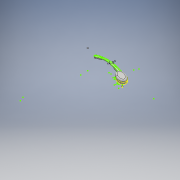
# Autodesk Inventor part: InnerPod
Saved by Autodesk Inventor 2016 (Build 200138000, 138)
## iProperties
Created: 2015-06-15
Part Number: InnerPod
Material: Generic
Document SubType Name: Modeling
Designer: Erin
Density: 1 g/cm^3
Appearance: Default
Author: Erin
Autodesk Inventor part; units mm, degrees
ref_plane "YZ Plane" through (0, 0, 0) normal (1, 0, 0) x (0, 1, 0)
sketch "Sketch1" plane through (0, 0, 0) normal (0, 0, 1) x (1, 0, 0)
  line L0 (0, -23.0647) -> (0, 59.7901) construction
  ellipse E0 centre (-14.0004, 12.1) end of major axis (-23.0535, 16.1357) minor radius 4.9157
  arc A0 (-24.1451, 19.8468) -> (-50.54, 25.9478) centre (-70.9085, -122.3194) ccw
  arc A1 (-29.3261, 18.5387) -> (-51.8244, 24.0854) centre (-73.9314, -113.9855) ccw
  arc A2 (-31.8925, 10.9139) -> (-44.4376, 12.262) centre (-55.0181, -145.2384) ccw
  arc A3 (-31.8925, 10.9139) -> (-26.6229, 7.7379) centre (-17.4265, 28.9559) ccw
  arc A4 (-24.9409, 14.9636) -> (-22.1909, 12.262) centre (-19.0136, 18.2468) ccw
  arc A5 (-26.6229, 7.7379) -> (-13.0654, 6.572) centre (-17.1508, 38.4743) ccw
  arc A6 (-24.9409, 14.9636) -> (-29.3261, 18.5387) centre (-31.8925, 10.9139) ccw
  arc A7 (-24.1451, 19.8468) -> (-17.2584, 18.0641) centre (-13.8815, 45.3013) ccw
  arc A8 (-50.54, 25.9478) -> (-75.3937, 22.2872) centre (-55.9595, -23.4584) ccw
  arc A9 (-75.3937, 22.2872) -> (-71.6688, 21.067) centre (-73.3522, 22.2238) ccw
  arc A10 (-51.8244, 24.0854) -> (-71.6688, 21.067) centre (-57.2432, -7.0315) ccw
  arc A11 (-75.3937, 22.2872) -> (-90.8007, 8.3693) centre (-63.623, -6.2295) ccw
  arc A12 (-44.4376, 12.262) -> (-65.1692, 5.2101) centre (-38.8966, -38.0273) ccw
  arc A13 (-69.6317, 5.2101) -> (-65.1692, 5.2101) centre (-67.4004, 17.1946) ccw
  arc A14 (-69.6317, 5.2101) -> (-86.7264, 2.9791) centre (-74.6345, -23.0647) ccw
  arc A15 (-91.0496, 2.5661) -> (-86.7264, 2.9791) centre (-89.7462, 11.7565) ccw
  arc A16 (-90.8007, 8.3693) -> (-91.0496, 2.5661) centre (-84.9194, 5.2101) ccw
  ellipse E1 centre (-14.0004, 12.1) end of major axis (-23.7436, 16.5326) minor radius 5.7074
  ellipse E2 centre (-14.0004, 12.1) end of major axis (-25.1676, 17.1231) minor radius 7.2205
  line L1 (-14.1688, 17.4082) -> (7.9431, 10.5495) construction
  line L2 (-13.9565, 18.1799) -> (8.2098, 11.3044) construction
  line L3 (-5.6332, 7.1546) -> (-15.3689, -1.2851) construction
  line L4 (-5.0965, 6.5612) -> (-14.2425, -1.3674) construction
  line L5 (-4.0088, 5.519) -> (-10.8447, -0.4071) construction
  line L6 (-13.3724, 19.5692) -> (7.8363, 12.9908) construction
  line L7 (-9.6767, 18.0114) -> (-18.3242, 6.1886)
  arc A17 (-50.3962, 27.1116) -> (-75.8521, 23.3664) centre (-55.9595, -23.4584) ccw
  arc A18 (-24.0317, 20.2324) -> (-17.2091, 18.461) centre (-13.8815, 45.3013) ccw
  arc A19 (-76.7002, 22.3279) -> (-70.8185, 20.0327) centre (-73.3522, 22.2238) ccw
  arc A20 (-52.04, 22.7961) -> (-70.8185, 20.0327) centre (-57.2432, -7.0315) ccw
  arc A21 (-25.2887, 14.7659) -> (-29.4537, 18.1596) centre (-31.8925, 10.9139) ccw
  arc A22 (-25.2887, 14.7659) -> (-22.3785, 11.9087) centre (-19.0136, 18.2468) ccw
  arc A23 (-26.8006, 7.3741) -> (-13.0146, 6.1752) centre (-17.1508, 38.4743) ccw
  arc A24 (-32.3718, 9.8038) -> (-44.4122, 11.0896) centre (-55.0181, -145.2384) ccw
  arc A25 (-44.4122, 11.0896) -> (-64.7397, 4.1038) centre (-38.8966, -38.0273) ccw
  arc A26 (-69.8402, 4.0608) -> (-64.7397, 4.1038) centre (-67.4004, 17.1946) ccw
  arc A27 (-69.8402, 4.0608) -> (-86.2871, 1.8952) centre (-74.6345, -23.0647) ccw
  arc A28 (-91.8404, 1.5181) -> (-86.2871, 1.8952) centre (-89.7462, 11.7565) ccw
  arc A29 (-91.8297, 8.9221) -> (-91.8404, 1.5181) centre (-84.9194, 5.2101) ccw
  arc A30 (-75.8393, 23.3669) -> (-91.8297, 8.9221) centre (-63.623, -6.2295) ccw
  line L8 (22.4734, 0) -> (-109.3623, 0) construction
  line L9 (0, 0) -> (-2, 0)
  line L10 (-2, 0) -> (-2, 2)
  line L11 (-2, 2) -> (0, 2)
  line L12 (0, 2) -> (0, 0)
  line L13 (-97, 32) -> (-95, 32)
  line L14 (-95, 32) -> (-95, 30)
  line L15 (-95, 30) -> (-97, 30)
  line L16 (-97, 30) -> (-97, 32)
  dimension "d9" = 0.8
  dimension "d11" = 0.8
  dimension "d14" = 1.5
  dimension "d16" = 1.5
  dimension "d21" = 0.4
  dimension "d22" = 0.4
  dimension "d23" = 0.4
  dimension "d64" = 2
  dimension "d65" = 2
  dimension "d66" = 2
  dimension "d67" = 2
  dimension "d68" = 30
  dimension "d69" = 95
  constraints: 62 point on circle, 34 end point, 31 centre point, 7 parallel, 4 horizontal, 2 perpendicular, 2 vertical, 35 other
  measures "d9" distance between parallel lines of L1 L2
  measures "d11" distance between parallel lines of L4 L3
  measures "d14" distance between parallel lines of L4 L5
  measures "d16" distance between parallel lines of L2 L6
  measures "d21" radial gap between concentric circles of A7 A18
  measures "d22" radial gap between concentric circles of A4 A22
  measures "d23" radial gap between concentric circles of A5 A23
  measures "d64" distance of L10.end L11.end
  measures "d65" distance of L9.end L10.end
  measures "d66" distance of L14.end L15.end
  measures "d67" distance of L13.end L14.end
  measures "d68" distance between parallel lines of L15 L8
  measures "d69" distance between parallel lines of L14 L0
extrude "Extrusion4" add sketch "Sketch1" along normal blind 6.4 contours E0 L7 | E0 A4 E1 A7 | E0 L7 E1 A4 | A7 E1 L7 E0 | L7 E0 | E0 A5 E1 L7 | E1 A22 A21 E2 A6 A4 | A4 A6 E2 A7 E1 | L7 E1 A5 E0 | A7 E2 A18 E1 | L7 A5 E2 A21 A22 E1 | E1 A5 L7 | L7 E2 A23 E1 | E1 A18 E2 L7 | E1 A23 E2 L7 A5 | L7 E2 A5
extrude "Extrusion5" cut sketch "Sketch1" along normal blind 5.4 contours E0 L7 | E0 A4 E1 A7 | E0 L7 E1 A4 | A7 E1 L7 E0 | L7 E0 | E0 A5 E1 L7 | L7 E1 A5 E0
sketch "Sketch3" plane through (0, 0, 0) normal (0, 0, 1) x (1, 0, 0)
  arc A0 (-22.4417, 19.646) -> (-19.6295, 18.8734) centre (-13.8815, 45.3013) ccw
  arc A1 (-25.2887, 14.7659) -> (-23.0979, 12.3467) centre (-19.0136, 18.2468) ccw
  arc A2 (-25.2887, 14.7659) -> (-25.5583, 15.1947) centre (-31.8925, 10.9139) ccw
  arc A3 (-17.8075, 5.9181) -> (-14.1373, 6.0512) centre (-17.1508, 38.4743) ccw
  ellipse E0 centre (-14.0004, 12.1) end of major axis (-25.1676, 17.1231) minor radius 7.2205 projected
  ellipse E1 centre (-14.0004, 12.1) end of major axis (-23.7436, 16.5326) minor radius 5.7074 projected
  ellipse E2 centre (-14.0004, 12.1) end of major axis (-4.2573, 7.6674) minor radius 5.7074 projected
  line L0 (-14.1321, 6.0475) -> (-18.4635, 9.206)
  line L1 (-18.4635, 9.206) -> (-23.0991, 12.3388)
  ellipse E3 centre (-14.0004, 12.1) end of major axis (-25.1676, 17.1231) minor radius 7.2205 projected
  line L2 (-17.805, 5.9169) -> (-22.6057, 8.0763)
  line L3 (-22.6057, 8.0763) -> (-25.7428, 12.7137)
  line L4 (-25.7428, 12.7137) -> (-25.5519, 15.1307)
  line L5 (-25.5519, 15.1307) -> (-25.9604, 19.264)
  line L6 (-25.9604, 19.264) -> (-22.42, 19.6483)
  line L7 (-23.0991, 12.3388) -> (-22.3785, 17.1974)
  line L8 (-22.3785, 17.1974) -> (-19.6698, 18.8691)
  point P0 (0, 0)
  constraints: 18 end point, 8 point on circle, 5 point on line, 4 centre point, 18 other
fillet "Fillet2" radius 2.6 1 edges at (-4.2573, 7.6674, 5.4)
fillet "Fillet3" radius 2.6 2 edges at (-3.2867, 6.2992, 6.4) (-24.7142, 17.9008, 6.4)
ref_plane "Work Plane1" through (0, 0, -1.95) normal (0, 0, 1) x (1, 0, 0)
ref_plane "Work Plane4" through (0, 0, 3.45) normal (0, 0, 1) x (1, 0, 0)
sketch "Sketch4" plane through (0, 0, 3.45) normal (0, 0, 1) x (1, 0, 0)
  arc A0 (-22.1175, 19.7708) -> (-49.8231, 26.3097) centre (-70.1916, -121.9576) ccw
  arc A1 (-49.8231, 26.3097) -> (-74.6768, 22.649) centre (-55.2426, -23.0966) ccw
  arc A2 (-74.6768, 22.649) -> (-70.9519, 21.4288) centre (-72.6353, 22.5856) ccw
  arc A3 (-45.6473, 23.4615) -> (-70.9519, 21.4288) centre (-55.7681, -9.0698) ccw
  arc A4 (-28.6092, 18.9005) -> (-45.6473, 23.4615) centre (-73.2145, -113.6237) ccw
  arc A5 (-22.7959, 14.7558) -> (-28.6092, 18.9005) centre (-32.2974, 7.5783) ccw
  ellipse E0 centre (2.1264, -8.7968) end of major axis (11.8695, -13.2294) minor radius 5.7074 (-3.5026, -2.0234) -> (-6.9816, -8.5428) ccw
  line L0 (-36.0635, 25.2992) -> (-37.0563, 21.4499)
  line L1 (-64.0289, 27.3464) -> (-63.2171, 24.1752)
  line L2 (-23.0267, 16.8944) -> (-20.6601, 15.8177)
  ellipse E1 centre (52.3036, 7.0335) end of major axis (-21.4673, 1.8982) minor radius 13.4866 (-17.6477, 6.6233) -> (-21.4417, 1.6763) ccw
  arc A6 (-18.3242, 6.1886) -> (-21.2408, 3.1571) centre (-16.8449, 1.8465) ccw
  arc A7 (-49.6368, 27.7981) -> (-74.2501, 24.4472) centre (-55.2426, -23.0966) ccw
  arc A8 (-19.2413, 20.3567) -> (-49.6368, 27.7981) centre (-70.1916, -121.9576) ccw
  arc A9 (-74.2501, 24.4472) -> (-74.6768, 22.649) centre (-72.6147, 23.1095) ccw
  ellipse E2 centre (-14.0004, 12.1) end of major axis (-25.1676, 17.1231) minor radius 7.2205 (-18.3242, 6.1886) -> (-18.3242, 6.1886) ccw
  arc A10 (-23.9725, 18.6979) -> (-18.3242, 6.1886) centre (-15.2772, 15.0942) ccw
  ellipse E3 centre (-14.0004, 12.1) end of major axis (-25.1676, 17.1231) minor radius 7.2205 projected
  arc A11 (-19.2413, 20.3567) -> (-25.1701, 17.1175) centre (-19.3411, 13.4938) ccw
  point P0 (0, 0)
  point P1 (-36.4382, 23.8463)
  point P2 (-63.6558, 25.8888)
  point P3 (-4.5271, -2.1925)
  point P4 (-7.4476, -7.6611)
  point P5 (-73.2711, 20.6446)
  point P6 (-7.9383, -1.0836)
  point P7 (-25.5531, 15.1871)
  dimension "d43" = 1.5
  constraints: 34 point on circle, 12 centre point, 6 end point, 2 point on line, 21 other
  measures "d43" radial gap between concentric circles of A0 A8
extrude "Extrusion19" add sketch "Sketch4" against normal blind 1.5 contours E2 A5 A4 L0 A0 | A11 A10 E2 | A0 L0 A8 A11 | L0 A4 A3 L1 A1 A0 | A0 A1 L1 A7 A8 L0 | A10 A11 E2 | L1 A3 A2 A1 | A1 A9 A7 L1 picked at (-23.0986, 19.2504) picked at (-24.3283, 18.252)
extrude "Extrusion20" add sketch "Sketch4" against normal blind 3 contours E2 A5 A4 L0 A0 | A11 A10 E2 | A0 L0 A8 A11 | A10 A11 E2 | L1 A3 A2 A1 | A1 A9 A7 L1 picked at (-23.0986, 19.2504) picked at (-24.3283, 18.252)
fillet "Fillet7" radius 3 4 edges at (-36.5599, 23.3745, 0.45) (-36.5599, 23.3745, 1.95) (-63.623, 25.7608, 0.45) (-63.623, 25.7608, 1.95)
extrude "Extrusion21" add sketch "Sketch1" along normal blind 0.3 contours L9 L10 L11 L12 | L13 L14 L15 L16
equation "\"d9\" = 2 * sp"
equation "\"d11\" = 2 * sp"
equation "\"d21\" = sp"
equation "\"d22\" = sp"
equation "\"d23\" = sp"
equation "\"d70\" = layer"
equation "\"layer\" = 0.3"
equation "\"sp\" = 0.4"
equation "\"sp_z\" = 0.15"
equation "\"d42\" = -6 * layer - sp_z"
body "Solid2"
